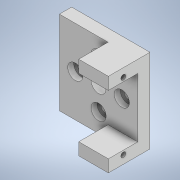
# Autodesk Inventor part: ServoESP32Base2
Saved by Autodesk Inventor 2020 (Build 240168000, 168)
## iProperties
Created: 2022-11-30
Part Number: ServoESP32Base2
Material: Generic
Document SubType Name: Modeling
Designer: agraa4529
Density: 1 g/cm^3
Appearance: Default
Author: agraa4529
## iProperties of the stored document _3DPrint.ipt
Created: 2022-12-02
Part Number: _3DPrint
Material: Generic
Document SubType Name: Modeling
Designer: agraa4529
Density: 1 g/cm^3
Appearance: Default
Author: agraa4529
Autodesk Inventor part; units mm, degrees
ref_plane "YZ Plane" through (0, 0, 0) normal (1, 0, 0) x (0, 1, 0)
ref_plane "XZ Plane" through (0, 0, 0) normal (0, 1, 0) x (-1, 0, 0)
ref_plane "XY Plane" through (0, 0, 0) normal (0, 0, 1) x (1, 0, 0)
sketch "Sketch1" plane through (0, 0, 0) normal (0, 0, 1) x (1, 0, 0)
  line L0 (-16, -16) -> (16, -16)
  line L1 (16, -16) -> (16, 16)
  line L2 (16, 16) -> (-16, 16)
  line L3 (-16, 16) -> (-16, -16)
  line L4 (-16, -16) -> (16, 16) construction
  line L5 (16, -16) -> (-16, 16) construction
  point P0 (0, 0)
  dimension "d1" = 32
  dimension "d2" = 32
  constraints: 12 end point, 2 midpoint, 2 parallel, 1 horizontal, 1 perpendicular
  measures "d1" distance of L2.end L1.end
  measures "d2" distance of L0.end L1.end
extrude "Extrusion1" add sketch "Sketch1" along normal blind 5
sketch "Sketch2" plane through (0, 0, 5) normal (0, 0, 1) x (1, 0, 0)
  line L0 (0, 0) -> (9.5, 0) construction
  circle A0 centre (9.5, 0) radius 1.5
  line L1 (0, 0) -> (0, 9.5) construction
  circle A1 centre (0, 9.5) radius 1.5
  line L2 (0, 0) -> (-9.5, 0) construction
  circle A2 centre (-9.5, 0) radius 1.5
  line L3 (0, 0) -> (0, -9.5) construction
  circle A3 centre (0, -9.5) radius 1.5
  dimension "d5" = 3
  dimension "d6" = 9.5
  dimension "d9" = 360
  constraints: 8 end point, 6 coincident, 4 centre point, 1 horizontal, 19 other
  measures "d5" diameter of A0
  measures "d6" distance of L0.start L0.end
extrude "Extrusion2" cut sketch "Sketch2" against normal blind 5
sketch "Sketch3" plane through (0, 0, 5) normal (0, 0, 1) x (1, 0, 0)
  circle A0 centre (0, 9.5) radius 1.5 projected
  circle A1 centre (0, 9.5) radius 3.1
  circle A2 centre (-9.5, 0) radius 3.1
  circle A3 centre (0, -9.5) radius 3.1
  circle A4 centre (9.5, 0) radius 3.1
  point P0 (0, 0)
  dimension "d13" = 6.2
  dimension "d16" = 360
  constraints: 4 centre point, 1 coincident, 9 other
  measures "d13" diameter of A1
extrude "Extrusion3" cut sketch "Sketch3" against normal blind 2.5
sketch "Sketch4" plane through (0, 0, 5) normal (0, 0, 1) x (1, 0, 0)
  line L0 (16, -16) -> (16, 16) projected
  line L1 (16, 0) -> (3.9, 0)
  line L2 (3.9, 0) -> (3.9, -12.1) construction
  line L3 (3.9, -12.1) -> (16, -12.1) construction
  line L4 (16, -12.1) -> (16, 0)
  line L5 (16, 0) -> (3.9, 0)
  line L6 (3.9, 0) -> (3.9, 12.1) construction
  line L7 (3.9, 12.1) -> (16, 12.1) construction
  line L8 (16, 12.1) -> (16, 0)
  line L9 (3.9, -12.1) -> (16, -12.1)
  line L10 (16, -12.1) -> (16, -17.1)
  line L11 (16, -17.1) -> (3.9, -17.1)
  line L12 (3.9, -17.1) -> (3.9, -12.1)
  line L13 (3.9, 12.1) -> (16, 12.1)
  line L14 (16, 12.1) -> (16, 17.1)
  line L15 (16, 17.1) -> (3.9, 17.1)
  line L16 (3.9, 17.1) -> (3.9, 12.1)
  point P0 (0, 0)
  point P1 (16, 12.1)
  point P2 (16, 16)
  dimension "d20" = 12.1
  dimension "d21" = 5
  dimension "d22" = 5
  dimension "d28" = 12.1
  dimension "d29" = 12.1
  constraints: 32 end point, 8 parallel, 4 horizontal, 4 perpendicular, 3 point on line, 1 midpoint
  measures "d20" distance of L3.end L2.end
  measures "d21" distance of L11.end L2.end
  measures "d22" distance of L15.end L6.end
  measures "d28" distance of L1.end L2.end
  measures "d29" distance of L5.end L6.end
extrude "Extrusion4" add sketch "Sketch4" along normal blind 12
sketch "Sketch5" plane through (0, 0, 5) normal (0, 0, 1) x (1, 0, 0)
  circle A0 centre (0, 0) radius 3
  dimension "d25" = 6
  constraints: 1 centre point, 1 coincident
  measures "d25" diameter of A0
extrude "Extrusion5" cut sketch "Sketch5" against normal blind 10
sketch "Sketch8" plane through (0, 0, 0) normal (0, 0, -1) x (-1, 0, 0)
  line L0 (16, -16) -> (-16, -16) projected
  line L1 (-16, -16) -> (16, -16)
  line L2 (16, -16) -> (16, -17.1)
  line L3 (16, -17.1) -> (-16, -17.1)
  line L4 (-16, -17.1) -> (-16, -16)
  line L5 (-16, 16) -> (16, 16) projected
  line L6 (-16, 16) -> (16, 16)
  line L7 (16, 16) -> (16, 17.1)
  line L8 (16, 17.1) -> (-16, 17.1)
  line L9 (-16, 17.1) -> (-16, 16)
  point P0 (0, 0)
  dimension "d30" = 32
  dimension "d31" = 1.1
  dimension "d32" = 32
  dimension "d33" = 1.1
  constraints: 16 end point, 4 parallel, 2 horizontal, 2 perpendicular
  measures "d30" distance of L2.end L3.end
  measures "d31" distance of L1.end L2.end
  measures "d32" distance of L7.end L8.end
  measures "d33" distance of L6.end L7.end
extrude "Extrusion6" add sketch "Sketch8" against normal blind 5
sketch "Sketch9" plane through (16, -17.1, 0) normal (1, 0, 0) x (0, 0, -1)
  line L0 (-5, 5) -> (-5, 0) projected
  line L1 (-5, 2.5) -> (-10.9, 2.5) construction
  line L2 (-10.9, 17.1) -> (-10.9, 3.4) construction
  circle A0 centre (-10.9, 3.4) radius 1
  line L3 (-10.9, 17.1) -> (-5, 17.1) construction
  line L4 (-5, 14.1) -> (-5, 20.1) projected
  circle A1 centre (-10.9, 30.8) radius 1
  point P0 (0, 17.1)
  dimension "d36" = 5.9
  dimension "d37" = 13.7
  dimension "d38" = 2
  constraints: 6 end point, 2 centre point, 2 midpoint, 1 coincident, 1 horizontal, 1 symmetric about line, 1 vertical, 1 other
  measures "d36" distance of L1.start L1.end
  measures "d37" distance of L2.start L2.end
  measures "d38" diameter of A0
extrude "Extrusion7" cut sketch "Sketch9" against normal blind 8
body "Solid1"
